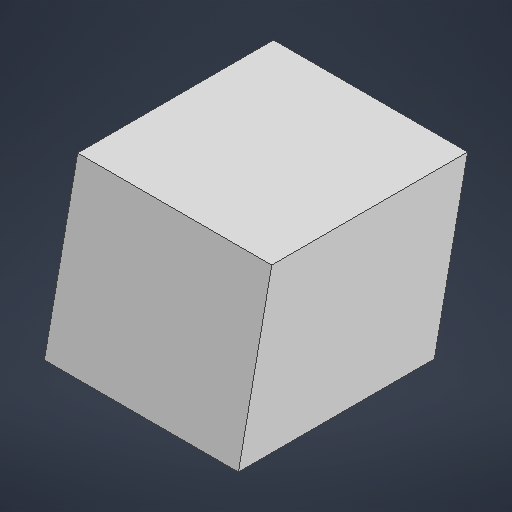
# Autodesk Inventor part: rod_v2.6
Saved by Autodesk Inventor 2026.2 (Build 302298000, 298)
## iProperties
Created: 2025-12-17
Part Number: rod_v2.6
Material: Generic
Document SubType Name: Modeling
Designer: Thoma
Density: 1 g/cm^3
Appearance: Default
Author: Thoma
Autodesk Inventor part; units mm, degrees
ref_plane "YZ Plane" through (0, 0, 0) normal (1, 0, 0) x (0, 1, 0)
ref_plane "XZ Plane" through (0, 0, 0) normal (0, 1, 0) x (-1, 0, 0)
ref_plane "XY Plane" through (0, 0, 0) normal (0, 0, 1) x (1, 0, 0)
sketch "Sketch2" plane through (0, 0, 0) normal (0, 0, 1) x (1, 0, 0)
  line L0 (-4.7, -6) -> (5.206, -6)
  line L1 (-3, 4) -> (6.906, 4)
  line L2 (-3, 4) -> (-4.7, -6)
  line L3 (6.906, 4) -> (5.206, -6)
  point P0 (0, 0)
  dimension "d4" = 9.906
  dimension "d5" = 9.906
  dimension "d6" = 1.7
  dimension "d7" = 10
  constraints: 8 end point, 1 horizontal
  measures "d4" distance of L0.start L0.end
  measures "d5" distance of L1.start L1.end
  measures "d6" horizontal distance of L0.start L1.start
  measures "d7" distance between parallel lines of L0 L1
extrude "Extrusion2" add sketch "Sketch2" along normal blind 10
body "Solid2"
